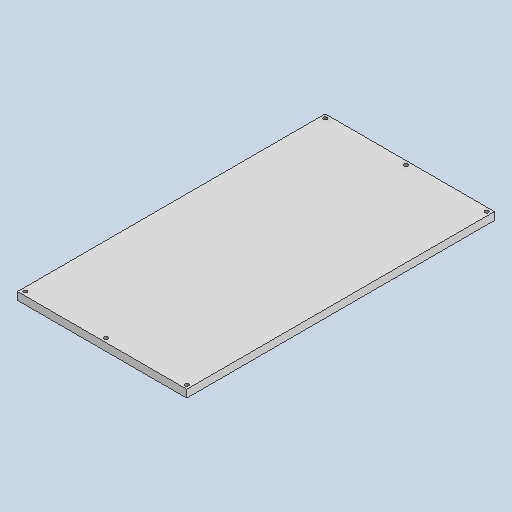
# Autodesk Inventor part: chassis_bas
Saved by Autodesk Inventor 2026.2 (Build 302298010, 298A)
## iProperties
Created: 2026-03-16
Part Number: chassis_bas
Material: Générique
Document SubType Name: Modeling
Designer: genon
Density: 1 g/cm^3
Appearance: Par défaut
Author: genon
Autodesk Inventor part; units mm, degrees
ref_plane "YZ Plane" through (0, 0, 0) normal (1, 0, 0) x (0, 1, 0)
ref_plane "XZ Plane" through (0, 0, 0) normal (0, 1, 0) x (-1, 0, 0)
ref_plane "XY Plane" through (0, 0, 0) normal (0, 0, 1) x (1, 0, 0)
sketch "Esquisse1" plane through (0, 0, 0) normal (0, 1, 0) x (-1, 0, 0)
  line L0 (55, -100) -> (-55, -100)
  line L1 (-55, -100) -> (-55, 100)
  line L2 (-55, 100) -> (55, 100)
  line L3 (55, 100) -> (55, -100)
  line L4 (55, -100) -> (-55, 100) construction
  line L5 (-55, -100) -> (55, 100) construction
  point P0 (0, 0)
  dimension "d0" = 110
  dimension "d1" = 200
  constraints: 12 end point, 2 midpoint, 2 parallel, 1 horizontal, 1 perpendicular
  measures "d0" distance of L1.end L2.end
  measures "d1" distance of L0.end L1.end
extrude "Extrusion1" add sketch "Esquisse1" along normal blind 5
sketch "Esquisse3" plane through (0, 0, 0) normal (0, -1, 0) x (1, 0, 0)
  line L0 (0, 0) -> (52.5, 0)
  line L1 (52.5, 0) -> (52.5, -97.5)
  line L2 (0, 28.6272) -> (0, -29.3855)
  point P0 (52.5, 97.5)
  point P1 (-52.5, -97.5)
  point P2 (-52.5, 97.5)
  dimension "d18" = 52.5
  dimension "d19" = 97.5
  constraints: 6 end point, 3 symmetric about line, 1 coincident, 1 horizontal, 1 perpendicular, 1 vertical
  measures "d18" distance of L0.start L0.end
  measures "d19" distance of L0.end L1.end
hole "Perçage2" at (52.5, 0, -97.5) at (52.5, 0, 97.5) at (-52.5, 0, -97.5) at (-52.5, 0, 97.5) direction (0, 1, 0) diameter 2.459 end through all thread size "M3x0.5" class "6H" standard "ISO Metric profile"
sketch "Esquisse4" plane through (0, 0, 0) normal (0, -1, 0) x (1, 0, 0)
  line L0 (0, 0) -> (0, 97.5)
  line L1 (0, 0) -> (87.5, 0)
  point P0 (0, -97.5)
  point P1 (-87.5, 0)
  dimension "d27" = 97.5
  dimension "d28" = 87.5
  constraints: 4 end point, 2 coincident, 2 symmetric about line, 1 horizontal, 1 vertical
  measures "d27" distance of L0.start L0.end
  measures "d28" distance of L0.start L1.end
hole "Perçage3" at (87.5, 0, 0) at (0, 0, 97.5) at (0, 0, -97.5) at (-87.5, 0, 0) direction (0, 1, 0) diameter 2.459 end through all thread size "M3x0.5" class "6H" standard "ISO Metric profile"
